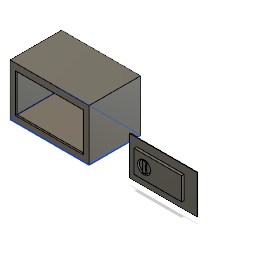
The Safe v2 (Autodesk Fusion 360 design; units mm, degrees)
Autodesk Fusion 360 part; units mm, degrees
sketch "Outer" plane through (0, 0, 0) normal (0, 1, 0) x (1, 0, 0)
  line L0 (-126.3687, 88.7654) -> (184.7813, 88.7654)
  line L1 (184.7813, 88.7654) -> (184.7813, -114.4346)
  line L2 (184.7813, -114.4346) -> (-126.3687, -114.4346)
  line L3 (-126.3687, -114.4346) -> (-126.3687, 88.7654)
  dimension "d2" = 311.15
  dimension "d3" = 203.2
  constraint horizontal L0
  constraint vertical L1
  constraint horizontal L2
  constraint vertical L3
  measures "d2" distance of L0.start L0.end
  measures "d3" distance of L0.start L2.end
extrude "Extrude1" add sketch "Outer" along normal blind 203.2 makes body 1
sketch "Inner" plane through (0, 0, 0) normal (0, 1, 0) x (1, 0, 0)
  line L0 (-123.1726, -108.4155) -> (181.6274, -108.4155)
  line L1 (181.6274, -108.4155) -> (181.6274, 82.0845)
  line L2 (181.6274, 82.0845) -> (-123.1726, 82.0845)
  line L3 (-123.1726, 82.0845) -> (-123.1726, -108.4155)
  dimension "d6" = 304.8
  dimension "d7" = 190.5
  constraint horizontal L0
  constraint vertical L1
  constraint horizontal L2
  constraint vertical L3
  measures "d6" distance of L0.start L0.end
  measures "d7" distance of L0.start L2.end
extrude "Extrude2" add sketch "Inner" along normal blind 177.8 separate body makes body 2
move_body "Move1" bodies 2 to x (1, 0, 0) y (0, 1, 0) z (0, 0, 1) at (0, 1, 0)
move_body "Move2" bodies 2 to x (1, 0, 0) y (0, 1, 0) z (0, 0, 1) at (0, 12.7, 0)
shell "Shell1" thickness 6.6 removed faces 0 bodies 1
sketch "Sketch4" plane through (0, 0, 114.4346) normal (0, 0, 1) x (1, 0, 0)
  line L0 (-126.3687, 0) -> (184.7813, 0)
  line L1 (184.7813, 0) -> (184.7813, 203.2)
  line L2 (184.7813, 203.2) -> (-126.3687, 203.2)
  line L3 (-126.3687, 203.2) -> (-126.3687, 0)
  line L4 (-104.5378, 176.7881) -> (162.1622, 176.7881)
  line L5 (162.1622, 176.7881) -> (162.1622, 24.3881)
  line L6 (162.1622, 24.3881) -> (-104.5378, 24.3881)
  line L7 (-104.5378, 24.3881) -> (-104.5378, 176.7881)
  dimension "d11" = 266.7
  dimension "d12" = 152.4
  constraint horizontal L4
  constraint vertical L5
  constraint horizontal L6
  constraint vertical L7
  measures "d11" distance of L4.start L4.end
  measures "d12" distance of L4.start L6.end
extrude "Extrude3" cut sketch "Sketch4" against normal blind 200 contours L4 L5 L6 L7 bodies 1 2
sketch "Sketch5" plane through (0, 0, 0) normal (0, 0, 1) x (1, 0, 0)
  line L0 (331.824, 176.4828) -> (598.524, 176.4828)
  line L1 (598.524, 176.4828) -> (598.524, 24.0828)
  line L2 (598.524, 24.0828) -> (331.824, 24.0828)
  line L3 (331.824, 24.0828) -> (331.824, 176.4828)
  dimension "d15" = 266.7
  dimension "d16" = 152.4
  constraint horizontal L0
  constraint vertical L1
  constraint horizontal L2
  constraint vertical L3
  measures "d15" distance of L0.start L0.end
  measures "d16" distance of L0.start L2.end
extrude "Extrude4" add sketch "Sketch5" along normal blind 3 separate body makes body 3
move_body "Move3" bodies 3 to x (1, 0, 0) y (0, 1, 0) z (0, 0, 1) at (0, 0, 100)
sketch "Sketch6" plane through (0, 0, 103) normal (0, 0, 1) x (1, 0, 0)
  line L0 (331.824, 24.0828) -> (598.524, 24.0828)
  line L1 (598.524, 24.0828) -> (598.524, 176.4828)
  line L2 (598.524, 176.4828) -> (331.824, 176.4828)
  line L3 (331.824, 176.4828) -> (331.824, 24.0828)
  line L4 (359.7261, 144.5625) -> (547.0461, 144.5625)
  line L5 (547.0461, 144.5625) -> (547.0461, 55.6625)
  line L6 (547.0461, 55.6625) -> (359.7261, 55.6625)
  line L7 (359.7261, 55.6625) -> (359.7261, 144.5625)
  dimension "d19" = 187.32
  dimension "d20" = 88.9
  constraint horizontal L4
  constraint vertical L5
  constraint horizontal L6
  constraint vertical L7
  measures "d19" distance of L4.start L4.end
  measures "d20" distance of L4.start L6.end
extrude "Extrude5" add sketch "Sketch6" along normal blind 10 contours L4 L5 L6 L7 bodies 3
sketch "Sketch7" plane through (0, 0, 113) normal (0, 0, 1) x (1, 0, 0)
  line L0 (359.7261, 55.6625) -> (547.0461, 55.6625)
  line L1 (547.0461, 55.6625) -> (547.0461, 144.5625)
  line L2 (547.0461, 144.5625) -> (359.7261, 144.5625)
  line L3 (359.7261, 144.5625) -> (359.7261, 55.6625)
  line L4 (484.6174, 138.4595) -> (538.5924, 138.4595)
  line L5 (538.5924, 138.4595) -> (538.5924, 60.672)
  line L6 (538.5924, 60.672) -> (484.6174, 60.672)
  line L7 (484.6174, 60.672) -> (484.6174, 138.4595)
  dimension "d23" = 53.975
  dimension "d24" = 77.7875
  constraint horizontal L4
  constraint vertical L5
  constraint horizontal L6
  constraint vertical L7
  measures "d23" distance of L4.start L4.end
  measures "d24" distance of L4.start L6.end
sketch "Sketch8" plane through (0, 0, 113) normal (0, 0, 1) x (1, 0, 0)
  line L0 (439.0755, 138.521) -> (474.0005, 138.521)
  line L1 (474.0005, 138.521) -> (474.0005, 60.7335)
  line L2 (474.0005, 60.7335) -> (439.0755, 60.7335)
  line L3 (439.0755, 60.7335) -> (439.0755, 138.521)
  line L4 (370.0653, 129.3511) -> (428.8008, 129.3511)
  line L5 (428.8008, 129.3511) -> (428.8008, 70.6156)
  line L6 (428.8008, 70.6156) -> (370.0653, 70.6156)
  line L7 (370.0653, 70.6156) -> (370.0653, 129.3511)
  dimension "d25" = 34.925
  dimension "d26" = 77.7875
  dimension "d27" = 58.7355
  dimension "d28" = 58.7355
  constraint horizontal L0
  constraint vertical L1
  constraint horizontal L2
  constraint vertical L3
  constraint horizontal L4
  constraint vertical L5
  constraint horizontal L6
  constraint vertical L7
  measures "d25" distance of L0.start L0.end
  measures "d26" distance of L0.start L2.end
  measures "d27" distance of L4.start L4.end
  measures "d28" distance of L4.start L6.end
sketch "Sketch9" plane through (0, 0, 113) normal (0, 0, 1) x (1, 0, 0)
  circle A0 centre (399.4799, 99.6431) radius 25.4
  dimension "d29" = 50.8
  measures "d29" diameter of A0
sketch "Sketch10" plane through (0, 0, 113) normal (0, 0, 1) x (1, 0, 0)
extrude "Extrude6" cut sketch "Sketch9" against normal blind 10 bodies 3
sketch "Sketch11" plane through (0, 0, 113) normal (0, 0, 1) x (1, 0, 0)
  circle A0 through (421.8377, 99.6517, -6) (388.0877, 119.1373, -6) (388.0877, 80.1661, -6)
extrude "Extrude7" add sketch "Sketch11" along normal blind 2 separate body contours A0 in plane through (0, 0, 107) normal (0, 0, 1) makes body 4
sketch "Sketch12" plane through (0, 0, 108) normal (0, 0, 1) x (1, 0, 0)
  line L0 (392.151, 120.8764) -> (407.8629, 120.8764)
  spline S0 degree 5 poles (392.151, 120.8764) (392.5491, 119.0642) (393.229, 115.4718) (393.9007, 110.1789) (394.196, 103.2868) (393.899, 94.8549) (393.3345, 88.1992) (392.7877, 83.2414) (392.3718, 79.9503) (392.151, 78.3082) knots 0 0 0 0 0 0 0.2 0.4 0.6 0.8 1 1 1 1 1 1
  spline S1 degree 5 poles (407.8629, 120.8764) (407.2998, 118.7129) (406.3379, 114.5267) (405.3877, 108.6698) (404.9701, 101.5886) (405.3902, 93.5447) (406.1888, 87.506) (406.9623, 83.1267) (407.5506, 80.2694) (407.8629, 78.8563) knots 0 0 0 0 0 0 0.2 0.4 0.6 0.8 1 1 1 1 1 1
  line L1 (407.8629, 78.8563) -> (392.151, 78.3082)
  line L2 (409.276, 126.3058) -> (406.4497, 115.447)
  line L3 (391.1477, 125.4442) -> (393.1544, 116.3085)
  constraint horizontal L0
  constraint midpoint L0.end L2
  constraint midpoint L0.start L3
extrude "Extrude8" add sketch "Sketch12" along normal blind 5 bodies 4
